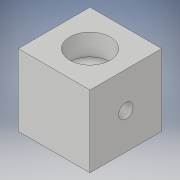
# Autodesk Inventor part: cubo_calibracion_tornillo_1cm
Saved by Autodesk Inventor 2019 (Build 230136000, 136)
## iProperties
Created: 2019-01-06
Part Number: cubo_calibracion_tornillo_1cm
Material: Generic
Document SubType Name: Modeling
Designer: assman
Density: 1 g/cm^3
Appearance: Default
Author: assman
Autodesk Inventor part; units mm, degrees
ref_plane "YZ Plane" through (0, 0, 0) normal (1, 0, 0) x (0, 1, 0)
ref_plane "XZ Plane" through (0, 0, 0) normal (0, 1, 0) x (-1, 0, 0)
ref_plane "XY Plane" through (0, 0, 0) normal (0, 0, 1) x (1, 0, 0)
sketch "Sketch1" plane through (0, 0, 0) normal (0, 1, 0) x (-1, 0, 0)
  line L0 (10, 0) -> (0, 0)
  line L1 (0, 0) -> (0, -10)
  line L2 (0, -10) -> (10, -10)
  line L3 (10, -10) -> (10, 0)
  dimension "d0" = 10
  dimension "d1" = 10
  constraints: 8 end point, 2 parallel, 1 coincident, 1 horizontal, 1 perpendicular
  measures "d0" distance of L2.end L1.end
  measures "d1" distance of L1.end L0.end
extrude "Extrusion1" add sketch "Sketch1" along normal blind 10
sketch "Sketch2" plane through (0, 10, 0) normal (0, 1, 0) x (1, 0, 0)
  line L0 (-10, 0) -> (0, 0) construction
  line L1 (0, 0) -> (0, 10) construction
  line L2 (0, 10) -> (-10, 10) construction
  line L3 (-10, 10) -> (-10, 0) construction
  circle A0 centre (-5, 5) radius 2.825
  dimension "d4" = 5.65
  constraints: 1 centre point
  measures "d4" diameter of A0
extrude "Extrusion2" cut sketch "Sketch2" against normal blind 3
sketch "Sketch3" plane through (-5, 7, -5) normal (0, 1, 0) x (1, 0, 0)
  circle A0 centre (0, 0) radius 1.425
  point P0 (5, -5)
  dimension "d7" = 2.85
  constraints: 1 centre point
  measures "d7" diameter of A0
extrude "Extrusion3" cut sketch "Sketch3" against normal through all
sketch "Sketch4" plane through (0, 0, 0) normal (1, 0, 0) x (0, 0, -1)
  line L0 (0, 0) -> (10, 0) construction
  line L1 (10, 0) -> (10, 10) construction
  line L2 (0, 10) -> (10, 10) construction
  line L3 (0, 0) -> (0, 10) construction
  circle A0 centre (5, 5) radius 1 construction
  circle A1 centre (5, 5) radius 1
  dimension "d10" = 2
  constraints: 2 centre point, 1 coincident, 1 concentric
  measures "d10" diameter of A0
extrude "Extrusion4" cut sketch "Sketch4" against normal blind 2
body "Solid1"
